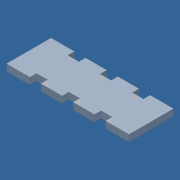
# Autodesk Inventor part: unionpress
Saved by Autodesk Inventor 2014 (Build 180170000, 170)
## iProperties
Created: 2013-09-11
Part Number: unionpress
Material: Glass
Document SubType Name: Modeling
Designer: Lefo
Density: 2.18 g/cm^3
Appearance: Clear
Author: Lefo
Autodesk Inventor part; units mm, degrees
ref_plane "YZ Plane" through (0, 0, 0) normal (1, 0, 0) x (0, 1, 0)
ref_plane "XZ Plane" through (0, 0, 0) normal (0, 1, 0) x (-1, 0, 0)
sketch "Sketch1" plane through (0, 0, 0) normal (0, 1, 0) x (-1, 0, 0)
  line L0 (0, 0) -> (-55, 0)
  line L1 (-55, 0) -> (-55, 20)
  line L2 (-55, 20) -> (0, 20)
  line L3 (0, 20) -> (0, 0)
  dimension "d0" = 55
  dimension "d1" = 20
  constraints: 8 end point, 2 parallel, 1 horizontal, 1 perpendicular
  measures "d0" distance of L1.end L2.end
  measures "d1" distance of L0.end L1.end
extrude "Extrusion1" add sketch "Sketch1" along normal blind 3
sketch "Sketch2" plane through (0, 3, 0) normal (0, 1, 0) x (1, 0, 0)
  line L0 (0, -20) -> (55, -20) projected
  line L1 (55, -20) -> (55, 0) projected
  line L2 (44.5, -20) -> (39.5, -20)
  line L3 (39.5, -20) -> (39.5, -17)
  line L4 (39.5, -17) -> (44.5, -17)
  line L5 (44.5, -17) -> (44.5, -20)
  line L6 (30, -20) -> (25, -20)
  line L7 (25, -20) -> (25, -17)
  line L8 (25, -17) -> (30, -17)
  line L9 (30, -17) -> (30, -20)
  line L10 (15.5, -20) -> (10.5, -20)
  line L11 (10.5, -20) -> (10.5, -17)
  line L12 (10.5, -17) -> (15.5, -17)
  line L13 (15.5, -17) -> (15.5, -20)
  point P0 (0, 0)
  dimension "d5" = 3
  dimension "d7" = 3
  dimension "d9" = 3
  dimension "d13" = 55
  dimension "d16" = 34
  dimension "d17" = 9.5
  dimension "d18" = 9.5
  dimension "d19" = 5
  dimension "d20" = 5
  dimension "d21" = 10.5
  constraints: 24 end point, 6 parallel, 3 horizontal, 3 perpendicular, 3 point on line
  measures "d5" distance of L2.end L3.end
  measures "d7" distance of L6.end L7.end
  measures "d9" distance of L10.end L11.end
  measures "d13" distance of L1.end point (0, 0)
  measures "d16" distance between parallel lines of L5 L11
  measures "d17" distance between parallel lines of L7 L13
  measures "d18" distance between parallel lines of L3 L9
  measures "d19" distance of L11.end L12.end
  measures "d20" distance of L7.end L8.end
  measures "d21" distance between parallel lines of L1 L5
extrude "Extrusion2" cut sketch "Sketch2" against normal blind 3
ref_plane "Work Plane1" through (55, 0, 10) normal (0, 0, 1) x (1, 0, 0)
mirror "Mirror1" about plane through (55, 0, 10) normal (0, 0, 1) of "Extrusion2"
equation "\"d18\" = d17"
equation "\"d20\" = d19"
equation "\"d21\" = -d17 + 0.5 * d13 - 1.5 * d19"
body "Solid1"
